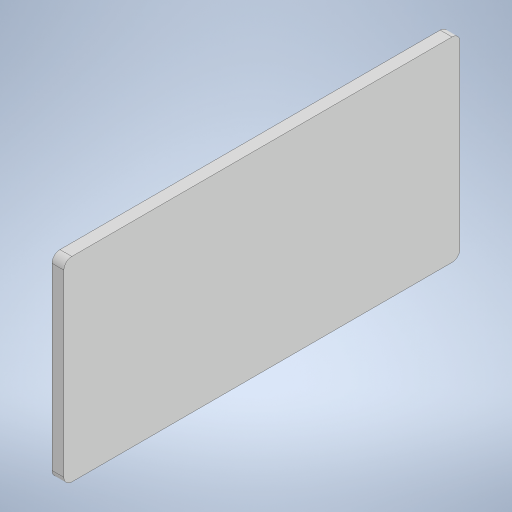
# Autodesk Inventor part: pokrywa_przod
Saved by Autodesk Inventor 2023 (Build 270158000, 158)
## iProperties
Created: 2024-07-28
Part Number: pokrywa_przod
Material: Ogólny
Document SubType Name: Modeling
Designer: kamil
Density: 1 g/cm^3
Appearance: Domyślna
Author: kamil
Autodesk Inventor part; units mm, degrees
ref_plane "YZ Plane" through (0, 0, 0) normal (1, 0, 0) x (0, 1, 0)
ref_plane "XZ Plane" through (0, 0, 0) normal (0, 1, 0) x (-1, 0, 0)
ref_plane "XY Plane" through (0, 0, 0) normal (0, 0, 1) x (1, 0, 0)
sketch "Szkic1" plane through (0, 0, 0) normal (1, 0, 0) x (0, 1, 0)
  line L0 (6.2889, 14.3259) -> (-43.0111, 14.3259)
  line L1 (-43.0111, 14.3259) -> (-43.0111, -85.6741)
  line L2 (-43.0111, -85.6741) -> (6.2889, -85.6741)
  line L3 (6.2889, -85.6741) -> (6.2889, 14.3259)
  point P0 (0, 0)
  dimension "d0" = 49.3
  dimension "d1" = 100
  constraints: 8 end point, 2 parallel, 1 horizontal, 1 perpendicular
  measures "d0" distance of L2.end L1.end
  measures "d1" distance of L1.end L0.end
extrude "Wyciągnięcie proste1" add sketch "Szkic1" along normal blind 3
fillet "Zaokrąglenie1" radius 2 4 edges at (1.5, 6.2889, 14.3259) (1.5, -43.0111, 14.3259) (1.5, 6.2889, -85.6741) (1.5, -43.0111, -85.6741)
